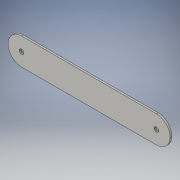
# Autodesk Inventor part: link
Saved by Autodesk Inventor 2016 (Build 200138000, 138)
## iProperties
Created: 2015-07-20
Part Number: link
Material: Generic
Document SubType Name: Modeling
Designer: chdsbd
Density: 1 g/cm^3
Appearance: Default
Author: chdsbd
Autodesk Inventor part; units mm, degrees
ref_plane "YZ Plane" through (0, 0, 0) normal (1, 0, 0) x (0, 1, 0)
ref_plane "XZ Plane" through (0, 0, 0) normal (0, 1, 0) x (-1, 0, 0)
ref_plane "XY Plane" through (0, 0, 0) normal (0, 0, 1) x (1, 0, 0)
sketch "Sketch1" plane through (0, 0, 0) normal (0, 0, 1) x (1, 0, 0)
  line L0 (0, 0) -> (190.5, 0) construction
  line L1 (0, -19.05) -> (190.5, -19.05)
  line L2 (190.5, 19.05) -> (0, 19.05)
  arc A0 (0, 19.05) -> (0, -19.05) centre (0, 0) ccw
  arc A1 (190.5, -19.05) -> (190.5, 19.05) centre (190.5, 0) ccw
  circle A2 centre (0, 0) radius 3.175
  circle A3 centre (190.5, 0) radius 3.175
  point P0 (95.25, 0)
  dimension "d0" = 190.5
  dimension "d1" = 38.1
  dimension "d2" = 6.35
  constraints: 8 end point, 4 centre point, 4 point on circle, 4 tangent, 2 coincident, 1 equal radius, 1 horizontal, 1 midpoint, 1 parallel
  measures "d0" distance of L0.start L0.end
  measures "d1" distance between parallel lines of L1 L2
  measures "d2" diameter of A2
extrude "Extrusion1" add sketch "Sketch1" along normal blind 2.54
body "Solid1"
